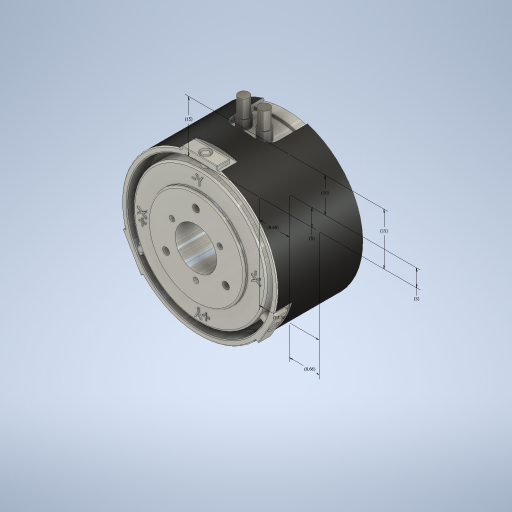
# Autodesk Inventor part: F6D45
Saved by Autodesk Inventor 2024 (Build 280153000, 153)
## iProperties
Created: 2023-03-02
Part Number: F6D45
Material: Acetal Resin, Black
Document SubType Name: Modeling
Designer: adars
Density: 1.425 g/cm^3
Appearance: Aluminum - Polished
Mass: 52.0581 g
Surface Area: 96.9356 cm^2
Volume: 36.532 cm^3
Author: adars
Autodesk Inventor part; units mm, degrees
ref_plane "YZ Plane" through (0, 0, 0) normal (1, 0, 0) x (0, 1, 0)
ref_plane "XY Plane" through (0, 0, 0) normal (0, 0, 1) x (1, 0, 0)
sketch "Sketch2" plane through (0, 0, 0) normal (0, 0, 1) x (1, 0, 0)
  circle A0 centre (0, 0) radius 14
  circle A1 centre (0, 0) radius 6
  dimension "d4" = 28
  dimension "d5" = 12
  constraints: 2 centre point, 2 coincident
  measures "d4" diameter of A0
  measures "d5" diameter of A1
extrude "Extrusion2" add sketch "Sketch2" along normal mid plane 27
fillet "Fillet1" radius 0.5 2 edges at (-14, 0, 13.5) (-14, 0, -13.5)
sketch "Sketch3" plane through (0, 0, 0) normal (0, 0, 1) x (1, 0, 0)
  circle A0 centre (0, 0) radius 22.5
  circle A1 centre (0, 0) radius 21
  dimension "d9" = 45
  dimension "d10" = 1.5
  constraints: 2 centre point, 1 coincident
  measures "d9" diameter of A0
  measures "d10" radial gap between concentric circles of A0 A1
extrude "Extrusion3" add sketch "Sketch3" along normal mid plane 25
fillet "Fillet2" radius 0.25 4 edges at (-21, 0, 12.5) (-22.5, 0, 12.5) (-22.5, 0, -12.5) (-21, 0, -12.5)
sketch "Sketch5" plane through (0, 0, 0) normal (0, 0, 1) x (1, 0, 0)
  circle A0 centre (0, 0) radius 14 projected
  circle A1 centre (0, 0) radius 21 projected
extrude "Extrusion5" add sketch "Sketch5" along normal mid plane 15
sketch "Sketch7" plane through (0, 0, 12.5) normal (0, 0, 1) x (1, 0, 0)
  line L0 (-6, 21.625) -> (6, 21.625)
  line L1 (6, 21.625) -> (6, 23.375)
  line L2 (6, 23.375) -> (-6, 23.375)
  line L3 (-6, 23.375) -> (-6, 21.625)
  line L4 (-6, 21.625) -> (6, 23.375) construction
  line L5 (6, 21.625) -> (-6, 23.375) construction
  circle A0 centre (0, 0) radius 6 projected
  circle A1 centre (0, 0) radius 13.5 projected
  circle A2 centre (0, 0) radius 6 projected
  line L6 (-15.7278, -16.0087) -> (-21.7278, -5.6163)
  line L7 (-21.7278, -5.6163) -> (-23.2433, -6.4913)
  line L8 (-23.2433, -6.4913) -> (-17.2433, -16.8837)
  line L9 (-17.2433, -16.8837) -> (-15.7278, -16.0087)
  line L10 (21.7278, -5.6163) -> (15.7278, -16.0087)
  line L11 (15.7278, -16.0087) -> (17.2433, -16.8837)
  line L12 (17.2433, -16.8837) -> (23.2433, -6.4913)
  line L13 (23.2433, -6.4913) -> (21.7278, -5.6163)
  point P0 (0, 22.5)
  point P1 (0, 22.5)
  point P2 (0, 22.5)
  dimension "d27" = 12
  dimension "d28" = 1.75
  dimension "d29" = 22.5
  dimension "d32" = 360
  constraints: 28 end point, 4 midpoint, 2 parallel, 1 horizontal, 1 perpendicular, 1 vertical alignment, 25 other
  measures "d27" distance of L0.start L0.end
  measures "d28" distance of L1.end L0.end
  measures "d29" distance of point (0, 0) point (0, 22.5)
extrude "Extrusion7" cut sketch "Sketch7" against normal blind 5 contours L3 L2 L1 L0 | L9 L8 L7 L6 | L13 L12 L11 L10
sketch "Sketch8" plane through (0, 0, 7.5) normal (0, 0, 1) x (1, 0, 0)
  circle A0 centre (0, 0) radius 19.25
  circle A1 centre (0, 0) radius 14
  dimension "d36" = 38.5
  dimension "d37" = 28
  constraints: 2 centre point, 2 coincident
  measures "d36" diameter of A0
  measures "d37" diameter of A1
extrude "Extrusion8" add sketch "Sketch8" along normal up to surface (5 mm away)
sketch "Sketch9" plane through (15.7278, -16.0087, 12.4102) normal (0.8660254, -0.5, 0) x (0, 0, -1)
  line L0 (-0.0898, 0.8335) -> (-0.0898, 11.1665)
  line L1 (-0.0898, 11.1665) -> (3.5102, 11.1665)
  line L2 (3.5102, 11.1665) -> (3.5102, 0.8335)
  line L3 (3.5102, 0.8335) -> (-0.0898, 0.8335)
  line L4 (-0.0898, 0.8335) -> (3.5102, 11.1665) construction
  line L5 (-0.0898, 11.1665) -> (3.5102, 0.8335) construction
  line L6 (4.9102, 0) -> (4.9102, 12) projected
  line L7 (4.9102, 0) -> (0.1602, 0) projected
  point P0 (12.4102, 6)
  point P1 (1.7102, 6)
  point P2 (1.7102, 6)
  dimension "d41" = 3.6
  dimension "d42" = 1.4
  dimension "d43" = 6
  dimension "d49" = 10.3331
  constraints: 12 end point, 3 midpoint, 2 parallel, 1 perpendicular, 1 vertical
  measures "d41" distance of L0.end L1.end
  measures "d42" distance between parallel lines of L2 L6
  measures "d43" distance from line of L7 point (1.71, 6)
  measures "d49" distance of L0.start L0.end
extrude "Extrusion9" add sketch "Sketch9" along normal blind 1
sketch "Sketch10" plane through (16.5938, -16.5087, 12.4102) normal (0.8660254, -0.5, 0) x (0, 0, -1)
  line L0 (3.5102, 11.1665) -> (-0.0898, 11.1665) projected
  line L1 (3.5102, 0.8335) -> (3.5102, 11.1665) projected
  line L2 (-0.0898, 0.8335) -> (3.5102, 0.8335) projected
  line L3 (-0.0898, 11.1665) -> (-0.0898, 0.8335) projected
  circle A0 centre (1.7102, 6) radius 1.5
  point P0 (12.4102, 6)
  dimension "d46" = 3
  dimension "d56" = 5.1665
  dimension "d57" = 1.8
  constraints: 1 centre point
  measures "d46" diameter of A0
  measures "d56" distance from line of L2 A0.centre
  measures "d57" distance from line of L3 A0.centre
extrude "Extrusion10" cut sketch "Sketch10" against normal blind 2.5 contours A0
sketch "Sketch11" plane through (-21.7278, -5.6163, 7.5) normal (-0.8660254, -0.5, 0) x (0, 0, 1)
  line L0 (1.4, -0.8335) -> (1.4, -11.1665)
  line L1 (1.4, -11.1665) -> (5, -11.1665)
  line L2 (5, -11.1665) -> (5, -0.8335)
  line L3 (5, -0.8335) -> (1.4, -0.8335)
  line L4 (1.4, -0.8335) -> (5, -11.1665) construction
  line L5 (1.4, -11.1665) -> (5, -0.8335) construction
  line L6 (0, 0) -> (4.75, 0) projected
  line L7 (0, 0) -> (0, -12) projected
  point P0 (-7.5, -6)
  point P1 (3.2, -6)
  point P2 (3.2, -6)
  dimension "d50" = 6
  dimension "d51" = 3.6
  dimension "d52" = 1.4
  dimension "d53" = 10.333
  constraints: 12 end point, 3 midpoint, 2 parallel, 1 perpendicular, 1 vertical
  measures "d50" distance from line of point (3.2, -6) L6
  measures "d51" distance of L0.end L1.end
  measures "d52" distance between parallel lines of L7 L0
  measures "d53" distance of L1.end L2.end
extrude "Extrusion11" add sketch "Sketch11" along normal blind 1
sketch "Sketch12" plane through (-22.5938, -6.1163, 7.5) normal (-0.8660254, -0.5, 0) x (0, 0, 1)
  circle A0 centre (3.2, -6) radius 1.5
  line L0 (5, -11.1665) -> (5, -0.8335) projected
  line L1 (5, -0.8335) -> (1.4, -0.8335) projected
  point P0 (-7.5, -6)
  dimension "d58" = 3
  dimension "d59" = 1.8
  dimension "d60" = 5.1665
  constraints: 1 centre point
  measures "d58" diameter of A0
  measures "d59" distance from line of L0 A0.centre
  measures "d60" distance from line of L1 A0.centre
extrude "Extrusion12" cut sketch "Sketch12" against normal blind 2
sketch "Sketch14" plane through (-5.2366, 21.625, 12.5) normal (0, 1, 0) x (1, 0, 0)
  line L0 (10.4031, 3.6) -> (0.0701, 3.6)
  line L1 (0.0701, 3.6) -> (0.0701, 0)
  line L2 (0.0701, 0) -> (10.4031, 0)
  line L3 (10.4031, 0) -> (10.4031, 3.6)
  line L4 (10.4031, 3.6) -> (0.0701, 0) construction
  line L5 (0.0701, 3.6) -> (10.4031, 0) construction
  line L6 (-0.7634, 0.25) -> (-0.7634, 5) projected
  line L7 (11.2366, 5) -> (-0.7634, 5) projected
  point P0 (5.2366, 12.5)
  point P1 (5.2366, 1.8)
  point P2 (5.2366, 1.8)
  dimension "d63" = 3.6
  dimension "d64" = 10.333
  dimension "d65" = 6
  dimension "d66" = 1.4
  constraints: 12 end point, 3 midpoint, 2 parallel, 1 horizontal, 1 perpendicular
  measures "d63" distance of L0.end L1.end
  measures "d64" distance of L0.start L0.end
  measures "d65" distance from line of L6 point (5.237, 1.8)
  measures "d66" distance between parallel lines of L7 L0
extrude "Extrusion13" add sketch "Sketch14" along normal blind 1
sketch "Sketch15" plane through (-5.2366, 22.625, 12.5) normal (0, 1, 0) x (1, 0, 0)
  circle A0 centre (5.2371, 1.8) radius 1.5
  line L0 (0.0701, 0) -> (10.4031, 0) projected
  line L1 (0.0701, 3.6) -> (0.0701, 0) projected
  point P0 (5.2366, 12.5)
  dimension "d69" = 3
  dimension "d70" = 1.8
  dimension "d71" = 5.167
  constraints: 1 centre point
  measures "d69" diameter of A0
  measures "d70" distance from line of L0 A0.centre
  measures "d71" distance from line of L1 A0.centre
extrude "Extrusion14" cut sketch "Sketch15" against normal blind 2
fillet "Fillet4" radius 0.15 23 edges at (-19.5938, -11.3125, 12.5) (-21.7441, -6.5882, 12.5) (-22.1771, -6.8382, 10.7) (-19.5938, -11.3125, 8.9) (-17.0106, -15.7868, 10.7) (-16.5776, -15.5368, 12.5) (-16.5776, -15.5368, 8.9) (-21.7441, -6.5882, 8.9) (-5.1665, 22.625, 10.7) (0, 22.625, 12.5) (0, 22.625, 8.9) (5.1665, 22.625, 10.7) (5.1665, 22.125, 12.5) (-5.1665, 22.125, 12.5) (5.1665, 22.125, 8.9) (-5.1665, 22.125, 8.9) (17.0106, -15.7869, 10.7) (16.5775, -15.5369, 12.5) (19.5938, -11.3125, 12.5) (19.5938, -11.3125, 8.9) (16.5775, -15.5369, 8.9) (22.1771, -6.8381, 10.7) (21.7441, -6.5881, 8.9)
sketch "Sketch16" plane through (16.5938, -16.5087, 12.4102) normal (0.8660254, -0.5, 0) x (0, 0, -1)
  circle A0 centre (1.7102, 6) radius 1.5 projected
  circle A1 centre (1.7102, 6) radius 1
  point P0 (12.4102, 6)
  dimension "d75" = 2
  constraints: 1 centre point, 1 coincident
  measures "d75" diameter of A1
extrude "Extrusion15" add sketch "Sketch16" against normal up to surface contours A1 round surface about axis through (0, 0, 7.5) along (0, 0, 1) radius 19.25 far side no
sketch "Sketch17" plane through (-5.2366, 22.625, 12.5) normal (0, 1, 0) x (1, 0, 0)
  circle A0 centre (5.2371, 1.8) radius 1.5 projected
  circle A1 centre (5.2371, 1.8) radius 1
  point P0 (5.2366, 12.5)
  dimension "d78" = 2
  constraints: 1 centre point, 1 coincident
  measures "d78" diameter of A1
extrude "Extrusion16" add sketch "Sketch17" against normal up to surface contours A1 round surface about axis through (0, 0, 7.5) along (0, 0, 1) radius 19.25 far side no
sketch "Sketch18" plane through (-22.5938, -6.1163, 7.5) normal (-0.8660254, -0.5, 0) x (0, 0, 1)
  circle A0 centre (3.2, -6) radius 1.5 projected
  circle A1 centre (3.2, -6) radius 1
  point P0 (-7.5, -6)
  dimension "d81" = 2
  constraints: 1 centre point, 1 coincident
  measures "d81" diameter of A1
extrude "Extrusion17" add sketch "Sketch18" against normal up to surface contours A1 round surface about axis through (0, 0, 7.5) along (0, 0, 1) radius 19.25 far side no
fillet "Fillet5" radius 0.15 3 edges at (-19.5938, -11.3125, 9.7) (-0.9995, 22.625, 10.7) (19.5938, -11.3125, 11.7)
fillet "Fillet6" radius 0.5 1 edges at (-19.25, 0, 12.5)
sketch "Sketch19" plane through (0, 0, 13.5) normal (0, 0, 1) x (1, 0, 0)
  circle A0 centre (0, 10) radius 1.25
  circle A1 centre (0, 0) radius 6 projected
  circle A2 centre (-8.6603, -5) radius 1.25
  circle A3 centre (8.6603, -5) radius 1.25
  dimension "d86" = 2.5
  dimension "d87" = 10
  dimension "d90" = 360
  constraints: 3 centre point, 1 vertical alignment, 7 other
  measures "d86" diameter of A0
  measures "d87" distance of point (0, 0) A0.centre
hole "Hole1" at (0, 10, 13.5) at (-8.6603, -5, 13.5) at (8.6603, -5, 13.5) direction (0, 0, -1) diameter 2.013 depth 8 tip angle 118 thread size "M2.5x0.45" class "6H" standard "ISO Metric profile"
sketch "Sketch20" plane through (0, 0, 13.5) normal (0, 0, 1) x (1, 0, 0)
  circle A0 centre (0, -8) radius 0.75
  circle A1 centre (0, 0) radius 6 projected
  circle A2 centre (6.9282, 4) radius 0.75
  circle A3 centre (-6.9282, 4) radius 0.75
  dimension "d99" = 1.5
  dimension "d100" = 8
  dimension "d103" = 360
  constraints: 3 centre point, 1 vertical alignment, 7 other
  measures "d99" diameter of A0
  measures "d100" distance of A0.centre point (0, 0)
hole "Hole2" at (0, -8, 13.5) at (6.9282, 4, 13.5) at (-6.9282, 4, 13.5) direction (0, 0, -1) diameter 1.5 depth 5
ref_plane "Work Plane1" through (0, 0, 17.5) normal (0, 0, 1) x (1, 0, 0)
sketch "Sketch21" plane through (0, 0, 17.5) normal (0, 0, 1) x (1, 0, 0)
  line L0 (-2.5, 18) -> (1.5, 18) construction
  line L1 (1.5, 18) -> (1.5, 15) construction
  line L2 (1.5, 15) -> (-2.5, 15) construction
  line L3 (-2.5, 15) -> (-2.5, 18) construction
  line L4 (18, 2.5) -> (18, -1.5) construction
  line L5 (18, -1.5) -> (15, -1.5) construction
  line L6 (15, -1.5) -> (15, 2.5) construction
  line L7 (15, 2.5) -> (18, 2.5) construction
  line L8 (-18, -3) -> (-18, 1) construction
  line L9 (-18, 1) -> (-15, 1) construction
  line L10 (-15, 1) -> (-15, -3) construction
  line L11 (-15, -3) -> (-18, -3) construction
  line L12 (3, -18) -> (-1, -18) construction
  line L13 (-1, -18) -> (-1, -15) construction
  line L14 (-1, -15) -> (3, -15) construction
  line L15 (3, -15) -> (3, -18) construction
  line L16 (-16.2057, -1.0103) -> (-16.2057, -1.8707)
  line L17 (-16.2057, -1.8707) -> (-15.3453, -1.8707)
  line L18 (-15.3453, -1.8707) -> (-15.3453, -2.1547)
  line L19 (-15.3453, -2.1547) -> (-16.2057, -2.1547)
  line L20 (-16.2057, -2.1547) -> (-16.2057, -3.0151)
  line L21 (-16.2057, -3.0151) -> (-16.4794, -3.0151)
  line L22 (-16.4794, -3.0151) -> (-16.4794, -2.1547)
  line L23 (-16.4794, -2.1547) -> (-17.3398, -2.1547)
  line L24 (-17.3398, -2.1547) -> (-17.3398, -1.8707)
  line L25 (-17.3398, -1.8707) -> (-16.4794, -1.8707)
  line L26 (-16.4794, -1.8707) -> (-16.4794, -1.0103)
  line L27 (-16.4794, -1.0103) -> (-16.2057, -1.0103)
  line L28 (-15.23, 1.2704) -> (-15.23, 0.8834)
  line L29 (-15.23, 0.8834) -> (-16.2427, 0.2659)
  line L30 (-16.2427, 0.2659) -> (-15.23, -0.364)
  line L31 (-15.23, -0.364) -> (-15.23, -0.7283)
  line L32 (-15.23, -0.7283) -> (-16.5021, 0.0806)
  line L33 (-16.5021, 0.0806) -> (-17.77, -0.7036)
  line L34 (-17.77, -0.7036) -> (-17.77, -0.3166)
  line L35 (-17.77, -0.3166) -> (-16.7758, 0.2885)
  line L36 (-16.7758, 0.2885) -> (-17.77, 0.906)
  line L37 (-17.77, 0.906) -> (-17.77, 1.2704)
  line L38 (-17.77, 1.2704) -> (-16.5185, 0.4758)
  line L39 (-16.5185, 0.4758) -> (-15.23, 1.2704)
  line L40 (-1.0455, 16.1871) -> (-2.0067, 16.1871)
  line L41 (-2.0067, 16.1871) -> (-2.0067, 16.4959)
  line L42 (-2.0067, 16.4959) -> (-1.0455, 16.4959)
  line L43 (-1.0455, 16.4959) -> (-1.0455, 16.1871)
  line L44 (1.1426, 17.77) -> (0.2842, 16.3539)
  line L45 (0.2842, 16.3539) -> (0.2842, 15.23)
  line L46 (0.2842, 15.23) -> (-0.0533, 15.23)
  line L47 (-0.0533, 15.23) -> (-0.0533, 16.3189)
  line L48 (-0.0533, 16.3189) -> (-0.9117, 17.77)
  line L49 (-0.9117, 17.77) -> (-0.5371, 17.77)
  line L50 (-0.5371, 17.77) -> (0.1175, 16.6523)
  line L51 (0.1175, 16.6523) -> (0.7844, 17.77)
  line L52 (0.7844, 17.77) -> (1.1426, 17.77)
  line L53 (16.1871, 1.0321) -> (16.1871, 1.9933)
  line L54 (16.1871, 1.9933) -> (16.4959, 1.9933)
  line L55 (16.4959, 1.9933) -> (16.4959, 1.0321)
  line L56 (16.4959, 1.0321) -> (16.1871, 1.0321)
  line L57 (15.23, -1.1333) -> (15.23, -0.7463)
  line L58 (15.23, -0.7463) -> (16.2427, -0.1288)
  line L59 (16.2427, -0.1288) -> (15.23, 0.501)
  line L60 (15.23, 0.501) -> (15.23, 0.8654)
  line L61 (15.23, 0.8654) -> (16.5021, 0.0564)
  line L62 (16.5021, 0.0564) -> (17.77, 0.8407)
  line L63 (17.77, 0.8407) -> (17.77, 0.4537)
  line L64 (17.77, 0.4537) -> (16.7758, -0.1515)
  line L65 (16.7758, -0.1515) -> (17.77, -0.769)
  line L66 (17.77, -0.769) -> (17.77, -1.1333)
  line L67 (17.77, -1.1333) -> (16.5185, -0.3388)
  line L68 (16.5185, -0.3388) -> (15.23, -1.1333)
  line L69 (1.0237, -16.4357) -> (1.8841, -16.4357)
  line L70 (1.8841, -16.4357) -> (1.8841, -15.5753)
  line L71 (1.8841, -15.5753) -> (2.1681, -15.5753)
  line L72 (2.1681, -15.5753) -> (2.1681, -16.4357)
  line L73 (2.1681, -16.4357) -> (3.0285, -16.4357)
  line L74 (3.0285, -16.4357) -> (3.0285, -16.7094)
  line L75 (3.0285, -16.7094) -> (2.1681, -16.7094)
  line L76 (2.1681, -16.7094) -> (2.1681, -17.5698)
  line L77 (2.1681, -17.5698) -> (1.8841, -17.5698)
  line L78 (1.8841, -17.5698) -> (1.8841, -16.7094)
  line L79 (1.8841, -16.7094) -> (1.0237, -16.7094)
  line L80 (1.0237, -16.7094) -> (1.0237, -16.4357)
  line L81 (-1.2796, -18) -> (-0.4213, -16.5839)
  line L82 (-0.4213, -16.5839) -> (-0.4213, -15.46)
  line L83 (-0.4213, -15.46) -> (-0.0837, -15.46)
  line L84 (-0.0837, -15.46) -> (-0.0837, -16.5489)
  line L85 (-0.0837, -16.5489) -> (0.7746, -18)
  line L86 (0.7746, -18) -> (0.4, -18)
  line L87 (0.4, -18) -> (-0.2546, -16.8823)
  line L88 (-0.2546, -16.8823) -> (-0.9215, -18)
  line L89 (-0.9215, -18) -> (-1.2796, -18)
  point P0 (0, 0)
  dimension "d113" = 4
  dimension "d114" = 3
  dimension "d115" = 2.5
  dimension "d116" = 15
  dimension "d117" = 3
  dimension "d118" = 4
  dimension "d119" = 15
  dimension "d120" = 2.5
  dimension "d123" = 3
  dimension "d124" = 4
  dimension "d125" = 15
  dimension "d126" = 3
  dimension "d127" = 4
  dimension "d128" = 3
  dimension "d129" = 15
  dimension "d130" = 3
  constraints: 8 other
  measures "d113" distance between parallel lines of L1 L3
  measures "d114" distance of L0.end L1.end
  measures "d115" distance from line of L3 point (0, 0)
  measures "d116" distance from line of point (0, 0) L2
  measures "d117" distance of L4.end L5.end
  measures "d118" distance of L4.start L4.end
  measures "d119" distance from line of point (0, 0) L6
  measures "d120" distance from line of point (0, 0) L7
  measures "d123" distance of L8.end L9.end
  measures "d124" distance of L8.start L8.end
  measures "d125" distance from line of point (0, 0) L10
  measures "d126" distance from line of point (0, 0) L11
  measures "d127" distance of L12.start L12.end
  measures "d128" distance of L14.end L12.start
  measures "d129" distance from line of point (0, 0) L14
  measures "d130" distance from line of point (0, 0) L15
emboss "Emboss1" sketch "Sketch21" operation add depth 0.25 direction (0, 0, -1)
sketch "Sketch23" plane through (0, 0, -12.5) normal (0, 0, -1) x (-1, 0, 0)
  circle A0 centre (0, 0) radius 6 projected
  arc A1 (6.0345, 20.1143) -> (-6.0345, 20.1143) centre (0, 0) ccw
  arc A2 (6.4655, 21.551) -> (-6.4655, 21.551) centre (0, 0) ccw
  circle A3 centre (0, 0) radius 21 projected
  line L0 (6.0345, 20.1143) -> (6.4655, 21.551)
  arc A4 (21.78, -5.6465) -> (6, 21.6852) centre (0, 0) ccw projected
  line L1 (-6.0345, 20.1143) -> (-6.4655, 21.551)
  arc A5 (-6, 21.6852) -> (-21.78, -5.6465) centre (0, 0) ccw projected
  point P0 (-6.25, 20.8327)
  point P1 (6.25, 20.8327)
  dimension "d135" = 1.5
  dimension "d136" = 1.5
  dimension "d137" = 12.5
  dimension "d138" = 6.25
  constraints: 8 point on circle, 4 end point, 2 centre point, 2 coincident, 2 midpoint
  measures "d135" distance of L0.start L0.end
  measures "d136" distance of L1.start L1.end
  measures "d137" distance of point (-6.25, 20.833) point (6.25, 20.833)
  measures "d138" horizontal distance of point (0, 0) point (6.25, 20.833)
extrude "Extrusion18" cut sketch "Sketch23" against normal blind 12.2 contours A1 L1 A2 L0
fillet "Fillet7" radius 3.5 2 edges at (-6.25, 20.8327, -0.3) (6.25, 20.8327, -0.3)
ref_plane "Work Plane2" through (0, 23.5, 0) normal (0, 1, 0) x (-1, 0, 0)
sketch "Sketch24" plane through (0, 23.5, 0) normal (0, 1, 0) x (-1, 0, 0)
  circle A0 centre (3, -3.3) radius 1.8
  circle A1 centre (-3, -3.3) radius 1.8
  line L0 (3.0344, -0.3) -> (-3.0344, -0.3) projected
  point P0 (0, 0)
  dimension "d143" = 3.6
  dimension "d144" = 3.6
  dimension "d145" = 6
  dimension "d146" = 3
  dimension "d147" = 3
  dimension "d148" = 3
  constraints: 2 centre point
  measures "d143" diameter of A0
  measures "d144" diameter of A1
  measures "d145" distance of A1.centre A0.centre
  measures "d146" horizontal distance of point (0, 0) A0.centre
  measures "d147" distance from line of L0 A0.centre
  measures "d148" distance from line of L0 A1.centre
extrude "Extrusion19" add sketch "Sketch24" against normal up to surface round surface about axis through (0, 0, -12.5) along (0, 0, 1) radius 21 far side no
sketch "Sketch25" plane through (0, 23.5, 0) normal (0, 1, 0) x (-1, 0, 0)
  circle A0 centre (3, -3.3) radius 1.8 projected
  circle A1 centre (-3, -3.3) radius 1.8 projected
  circle A2 centre (3, -3.3) radius 1.5
  circle A3 centre (-3, -3.3) radius 1.5
  point P0 (0, 0)
  dimension "d151" = 3
  dimension "d152" = 3
  constraints: 2 centre point, 2 coincident
  measures "d151" diameter of A2
  measures "d152" diameter of A3
extrude "Extrusion20" add sketch "Sketch25" along normal blind 5 contours A2 | A3
sketch "Sketch26" plane through (0, 0, -7.5) normal (0, 0, -1) x (-1, 0, 0)
  arc A0 (-6.0345, 20.1143) -> (6.0345, 20.1143) centre (0, 0) ccw projected
  circle A1 centre (0, 0) radius 14 projected
  circle A2 centre (0, 0) radius 21
  circle A3 centre (0, 0) radius 14
  point P0 (6.0345, 20.1143)
  point P1 (-6.0345, 20.1143)
  constraints: 2 centre point, 2 coincident, 1 concentric
extrude "Extrusion21" add sketch "Sketch26" along normal blind 2
sketch "Sketch27" plane through (0, 0, -9.5) normal (0, 0, -1) x (-1, 0, 0)
  circle A0 centre (0, 0) radius 21.75
  circle A1 centre (0, 0) radius 21
  dimension "d157" = 43.5
  dimension "d158" = 42
  constraints: 2 centre point, 2 coincident
  measures "d157" diameter of A0
  measures "d158" diameter of A1
extrude "Extrusion22" cut sketch "Sketch27" along normal blind 10
sketch "Sketch28" plane through (0, 0, -9.5) normal (0, 0, -1) x (-1, 0, 0)
  circle A0 centre (0, 0) radius 14
  circle A1 centre (0, 0) radius 21.75
  constraints: 2 centre point, 2 coincident
fillet "Fillet8" radius 0.25 1 edges at (0, -21.75, -12.5)
extrude "Extrusion23" add sketch "Sketch28" along normal up to surface (3 mm away)
sketch "Sketch29" plane through (0, 0, -13.5) normal (0, 0, -1) x (-1, 0, 0)
  circle A0 centre (0, 10) radius 1.0065 projected
  circle A1 centre (0, 10) radius 1.25
  circle A2 centre (0, 0) radius 6 projected
  circle A3 centre (-8.6603, -5) radius 1.25
  circle A4 centre (8.6603, -5) radius 1.25
  dimension "d165" = 2.5
  dimension "d166" = 10
  dimension "d169" = 360
  constraints: 3 centre point, 1 vertical alignment, 7 other
  measures "d165" diameter of A1
  measures "d166" distance of point (0, 0) A1.centre
hole "Hole3" at (-8.6603, -5, -13.5) at (8.6603, -5, -13.5) at (0, 10, -13.5) direction (0, 0, 1) diameter 2.013 depth 8 tip angle 118 thread size "M2.5x0.45" class "6H" standard "ISO Metric profile"
sketch "Sketch30" plane through (0, 0, -13.5) normal (0, 0, -1) x (-1, 0, 0)
  circle A0 centre (0, -8) radius 0.75
  circle A1 centre (0, 0) radius 6 projected
  circle A2 centre (0, -8) radius 0.75 projected
  circle A3 centre (6.9282, 4) radius 0.75
  circle A4 centre (-6.9282, 4) radius 0.75
  dimension "d178" = 1.5
  dimension "d179" = 8
  dimension "d182" = 360
  constraints: 3 centre point, 1 vertical alignment, 7 other
  measures "d178" diameter of A0
  measures "d179" distance of point (0, 0) A0.centre
hole "Hole4" at (0, -8, -13.5) at (6.9282, 4, -13.5) at (-6.9282, 4, -13.5) direction (0, 0, 1) diameter 1.5 depth 5
sketch "Sketch31" plane through (0, 0, -13.5) normal (0, 0, -1) x (-1, 0, 0)
  circle A0 centre (8.6603, -5) radius 1.0065 projected
  circle A1 centre (0, 10) radius 1.0065 projected
  circle A2 centre (-8.6603, -5) radius 1.0065 projected
  point P0 (0, 0)
  dimension "d191" = 15
  dimension "d192" = 15
  dimension "d193" = 17.3205
  dimension "d194" = 10
  dimension "d195" = 8.6602
  dimension "d196" = 5
  dimension "d197" = 8.6602
  dimension "d198" = 5
  measures "d191" vertical distance of A0.centre A1.centre
  measures "d192" vertical distance of A1.centre A2.centre
  measures "d193" distance of A0.centre A2.centre
  measures "d194" distance of A1.centre point (0, 0)
  measures "d195" horizontal distance of A0.centre point (0, 0)
  measures "d196" vertical distance of A0.centre point (0, 0)
  measures "d197" horizontal distance of A2.centre point (0, 0)
  measures "d198" vertical distance of A2.centre point (0, 0)
body "Solid2"
